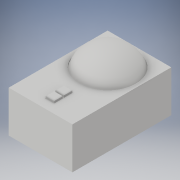
# Autodesk Inventor part: mouse ball
Saved by Autodesk Inventor 2017 (Build 210142000, 142)
## iProperties
Created: 2018-03-13
Part Number: mouse ball
Material: Generic
Document SubType Name: Modeling
Designer: Braxton
Density: 1 g/cm^3
Appearance: Default
Author: Braxton
Autodesk Inventor part; units mm, degrees
ref_plane "YZ Plane" through (0, 0, 0) normal (1, 0, 0) x (0, 1, 0)
ref_plane "XZ Plane" through (0, 0, 0) normal (0, 1, 0) x (-1, 0, 0)
ref_plane "XY Plane" through (0, 0, 0) normal (0, 0, 1) x (1, 0, 0)
sketch "Sketch1" plane through (0, 0, 0) normal (1, 0, 0) x (0, 1, 0)
  arc A0 (38.9763, 0) -> (-38.9763, 0) centre (0, 0) ccw
  arc A1 (42.4307, 0) -> (-42.4307, 0) centre (0, 0) ccw
  line L0 (-45.8851, 0) -> (-45.8851, 45.8851)
  line L1 (13.8845, 45.8851) -> (-45.8851, 45.8851)
  line L2 (13.8845, 45.8851) -> (13.8845, 0)
  line L3 (-45.8851, 0) -> (-45.8851, -45.8851)
  line L4 (13.8845, -45.8851) -> (-45.8851, -45.8851)
  line L5 (13.8845, -45.8851) -> (13.8845, 0)
  line L6 (42.9387, 0) -> (42.4307, 0)
  line L7 (38.9763, 0) -> (42.4307, 0)
  line L8 (38.9763, 0) -> (-38.9763, 0)
  line L9 (-38.9763, 0) -> (-42.4307, 0)
  line L10 (-42.4307, 0) -> (-42.9387, 0)
  dimension "d0" = 77.9526
  dimension "d3" = 45.8851
  dimension "d4" = 45.8851
  dimension "d10" = 3.4544
  dimension "d19" = 91.7702
  constraints: 22 end point, 4 point on circle, 3 collinear, 2 centre point, 2 coincident, 2 perpendicular, 1 horizontal, 1 other
  measures "d0" diameter of A0
  measures "d3" distance from line of A1.centre L1
  measures "d4" distance from line of L0 A1.centre
  measures "d10" radial gap between concentric circles of A0 A1
  measures "d19" distance between parallel lines of L4 L1
extrude "cube to cut from" add sketch "Sketch1" along normal mid plane 91.7702 contours L2 L8 A0 | A0 L9 A1 L2 | L5 L4 L3 L0 L1 L2 A1 L9 L8 picked at (-21.0569, 2.7719)
sketch "Sketch2" plane through (0, 0, 0) normal (1, 0, 0) x (0, 1, 0)
  arc A0 (42.9387, 0) -> (-42.9387, 0) centre (0, 0) ccw
  line L0 (42.9387, 0) -> (-42.9387, 0)
  dimension "d17" = 85.8774
  constraints: 2 end point, 2 point on circle, 1 centre point, 1 coincident, 1 horizontal
  measures "d17" diameter of A0
revolve "cut out for mouse ball" cut sketch "Sketch2" angle 360 about axis through (0, 42.9387, 0) along (0, -1, 0)
revolve "mouse ball" add sketch "Sketch1" angle 360 about axis through (0, 38.9763, 0) along (0, -1, 0) separate body contours A0 L2 A1 L7 | A0 L9 A1 L2
sketch "Sketch3" plane through (-45.8851, -45.8851, 45.8851) normal (0, 0, 1) x (1, 0, 0)
  line L0 (0, 59.7696) -> (91.7702, 59.7696) projected
  line L1 (0, 59.7696) -> (91.7702, 59.7696)
  line L2 (91.7702, 59.7696) -> (91.7702, 0) projected
  line L3 (91.7702, 59.7696) -> (91.7702, 0)
  line L4 (0, 0) -> (91.7702, 0) projected
  line L5 (91.7702, 0) -> (0, 0)
  line L6 (0, 0) -> (0, 59.7696)
  point P0 (45.8851, 45.8851)
  constraints: 8 end point, 2 collinear, 2 perpendicular
extrude "extention" add sketch "Sketch3" along normal blind 50.8 bodies 1
sketch "Sketch4" plane through (-45.8851, 13.8845, 96.6851) normal (0, 1, 0) x (1, 0, 0)
  line L0 (39.2811, 13.0556) -> (52.4891, 13.0556)
  line L1 (52.4891, 13.0556) -> (52.4891, 26.2636)
  line L2 (52.4891, 26.2636) -> (39.2811, 26.2636)
  line L3 (39.2811, 26.2636) -> (39.2811, 13.0556)
  circle A0 centre (45.8851, 96.6851) radius 42.9387 projected
  line L4 (45.8851, 53.7464) -> (45.8851, 0) construction
  line L5 (91.7702, 0) -> (0, 0) projected
  line L6 (39.2811, 40.3098) -> (52.4891, 40.3098)
  line L7 (52.4891, 40.3098) -> (52.4891, 27.1018)
  line L8 (52.4891, 27.1018) -> (39.2811, 27.1018)
  line L9 (39.2811, 27.1018) -> (39.2811, 40.3098)
  point P0 (45.8851, 26.2636)
  point P1 (39.2811, 19.6596)
  point P2 (45.8851, 40.3098)
  dimension "d23" = 13.208
  dimension "d24" = 13.208
  dimension "d39" = 53.7464
  dimension "d40" = 13.208
  dimension "d41" = 13.208
  dimension "d42" = 13.4366
  dimension "d47" = 0.8382
  constraints: 18 end point, 4 midpoint, 4 parallel, 2 horizontal, 2 perpendicular, 2 point on line, 1 vertical alignment, 1 other
  measures "d23" distance of L2.end L0.start
  measures "d24" distance of L1.end L2.end
  measures "d39" distance of L4.start L4.end
  measures "d40" distance of L8.end L6.start
  measures "d41" distance of L6.start L6.end
  measures "d42" distance of L4.start point (45.885, 40.31)
  measures "d47" distance between parallel lines of L2 L8
extrude "button hole" cut sketch "Sketch4" against normal blind 2.54 contours L3 L2 L1 L0 | L6 L7 L8 L9 bodies 1
ref_plane "button in hole" through (-45.8851, 12.6145, -45.8851) normal (0, 1, 0) x (1, 0, 0)
sketch "Sketch5" plane through (-45.8851, 12.6145, -45.8851) normal (0, 1, 0) x (1, 0, 0)
  line L0 (39.2811, -129.5146) -> (39.2811, -116.3066)
  line L1 (39.2811, -116.3066) -> (52.4891, -116.3066)
  line L2 (39.2811, -129.5146) -> (39.2811, -116.3066)
  line L3 (39.2811, -116.3066) -> (52.4891, -116.3066)
  line L4 (52.4891, -129.5146) -> (39.2811, -129.5146)
  line L5 (52.4891, -116.3066) -> (52.4891, -129.5146)
  line L6 (52.4891, -129.5146) -> (39.2811, -129.5146)
  line L7 (39.7891, -129.0066) -> (51.9811, -129.0066)
  line L8 (51.9811, -129.0066) -> (51.9811, -116.8146)
  line L9 (51.9811, -116.8146) -> (39.7891, -116.8146)
  line L10 (39.7891, -116.8146) -> (39.7891, -129.0066)
  line L11 (39.2811, -116.3066) -> (52.4891, -116.3066) projected
  line L12 (39.2811, -102.2604) -> (52.4891, -102.2604) projected
  line L13 (39.2811, -115.4684) -> (39.2811, -102.2604)
  line L14 (39.2811, -102.2604) -> (52.4891, -102.2604)
  line L15 (39.2811, -115.4684) -> (39.2811, -102.2604)
  line L16 (39.2811, -102.2604) -> (52.4891, -102.2604)
  line L17 (52.4891, -115.4684) -> (39.2811, -115.4684)
  line L18 (52.4891, -102.2604) -> (52.4891, -115.4684)
  line L19 (52.4891, -115.4684) -> (39.2811, -115.4684)
  line L20 (39.7891, -114.9604) -> (51.9811, -114.9604)
  line L21 (51.9811, -114.9604) -> (51.9811, -102.7684)
  line L22 (51.9811, -102.7684) -> (39.7891, -102.7684)
  line L23 (39.7891, -102.7684) -> (39.7891, -114.9604)
  point P0 (45.8851, -45.8851)
  dimension "d30" = 0.508
  dimension "d31" = 0.508
  dimension "d32" = 0.508
  dimension "d33" = 0.508
  dimension "d43" = 0.508
  dimension "d44" = 0.508
  dimension "d45" = 0.508
  dimension "d46" = 0.508
  constraints: 44 end point, 8 perpendicular, 6 equal length, 2 horizontal
  measures "d30" distance between parallel lines of L0 L10
  measures "d31" distance between parallel lines of L1 L9
  measures "d32" distance between parallel lines of L5 L8
  measures "d33" distance between parallel lines of L4 L7
  measures "d43" distance between parallel lines of L13 L23
  measures "d44" distance between parallel lines of L14 L22
  measures "d45" distance between parallel lines of L18 L21
  measures "d46" distance between parallel lines of L17 L20
extrude "button" add sketch "Sketch5" along normal blind 3.81 separate body contours L10 L9 L8 L7 | L23 L22 L21 L20
equation "\"d3\" = 0.5 * d0 + 2 * d1"
equation "\"d4\" = 0.5 * d0 + 2 * d1"
equation "\"d8\" = d19"
equation "\"d17\" = 2 * d10 + d0 + 2 * d11"
equation "\"d24\" = d23"
equation "\"d40\" = d23"
equation "\"d41\" = d23"
equation "\"d42\" = 0.25 * d39"
equation "\"d31\" = d30"
equation "\"d32\" = d30"
equation "\"d33\" = d30"
equation "\"d44\" = d43"
equation "\"d45\" = d43"
equation "\"d46\" = d43"
equation "\"d1\" = 3.4544"
equation "\"d11\" = 0.508"
